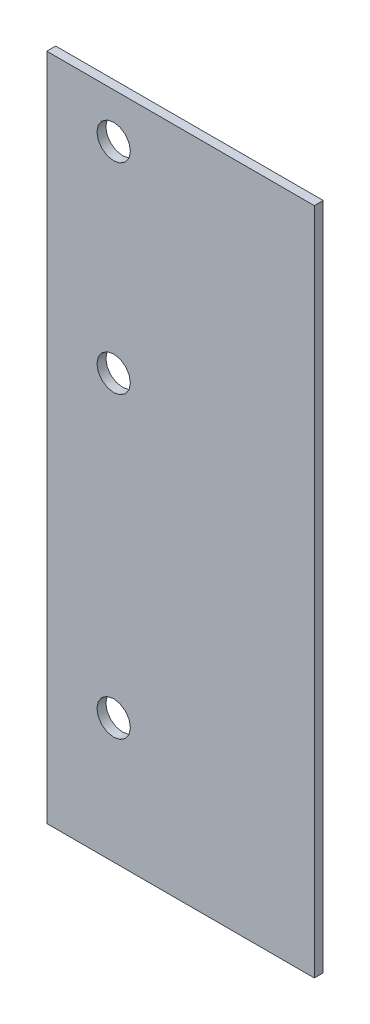
# Autodesk Inventor part: gabarito-suporte-motor-embaixo
Saved by Autodesk Inventor 2017 (Build 210142000, 142)
## iProperties
Created: 2018-08-18
Part Number: gabarito-suporte-motor-embaixo
Material: Wood (Oak)
Document SubType Name: Sheet Metal
Designer: Luiz Gustavo
Density: 0.76 g/cm^3
Sheet Metal Rule: Default_mm
Appearance: White Oak - Natural Medium Gloss
Author: Luiz Gustavo
Autodesk Inventor part; units mm, degrees
ref_plane "YZ Plane" through (0, 0, 0) normal (1, 0, 0) x (0, 1, 0)
ref_plane "XZ Plane" through (0, 0, 0) normal (0, 1, 0) x (-1, 0, 0)
ref_plane "XY Plane" through (0, 0, 0) normal (0, 0, 1) x (1, 0, 0)
sketch "Sketch1" plane through (0, 0, 0) normal (0, 0, 1) x (1, 0, 0)
  line L0 (16.1981, 153.4586) -> (16.9799, 152.4795) construction
  arc A0 (16.1981, 153.4586) -> (16.1981, 156.4471) centre (13, 154.9529) ccw construction
  line L1 (16.9799, 157.4262) -> (16.1981, 156.4471) construction
  arc A1 (16.9799, 157.4262) -> (15.4733, 158.9328) centre (16.1422, 158.0951) ccw construction
  line L2 (14.4942, 158.151) -> (15.4733, 158.9328) construction
  arc A2 (14.4942, 158.151) -> (11.5058, 158.151) centre (13, 154.9529) ccw construction
  line L3 (10.5267, 158.9328) -> (11.5058, 158.151) construction
  arc A3 (10.5267, 158.9328) -> (9.0201, 157.4262) centre (9.8578, 158.0951) ccw construction
  line L4 (9.8019, 156.4471) -> (9.0201, 157.4262) construction
  arc A4 (9.8019, 156.4471) -> (9.8019, 153.4586) centre (13, 154.9529) ccw construction
  line L5 (9.0201, 152.4795) -> (9.8019, 153.4586) construction
  arc A5 (9.0201, 152.4795) -> (10.5267, 150.9729) centre (9.8578, 151.8106) ccw construction
  line L6 (11.5058, 151.7547) -> (10.5267, 150.9729) construction
  arc A6 (11.5058, 151.7547) -> (14.4942, 151.7547) centre (13, 154.9529) ccw construction
  line L7 (15.4733, 150.9729) -> (14.4942, 151.7547) construction
  arc A7 (15.4733, 150.9729) -> (16.9799, 152.4795) centre (16.1422, 151.8106) ccw construction
  line L8 (26.6999, 145.0719) -> (26.6999, 142.2529) construction
  arc A8 (26.6999, 145.0719) -> (26.319, 145.4529) centre (26.319, 145.0719) ccw construction
  line L9 (22.88, 145.4529) -> (26.319, 145.4529) construction
  arc A9 (22.88, 145.4529) -> (22.5, 145.0729) centre (22.88, 145.0729) ccw construction
  line L10 (22.5, 141.6339) -> (22.5, 145.0729) construction
  arc A10 (22.5, 141.6339) -> (22.881, 141.2529) centre (22.881, 141.6339) ccw construction
  line L11 (25.7, 141.2529) -> (22.881, 141.2529) construction
  arc A11 (25.7, 141.2529) -> (26.6999, 142.2529) centre (25.7, 142.2529) ccw construction
  line L12 (-0.6999, 164.8338) -> (-0.6999, 167.6528) construction
  arc A12 (-0.6999, 164.8338) -> (-0.3189, 164.4528) centre (-0.3189, 164.8338) ccw construction
  line L13 (3.12, 164.4528) -> (-0.3189, 164.4528) construction
  arc A13 (3.12, 164.4528) -> (3.5, 164.8328) centre (3.12, 164.8328) ccw construction
  line L14 (3.5, 168.2718) -> (3.5, 164.8328) construction
  arc A14 (3.5, 168.2718) -> (3.119, 168.6528) centre (3.119, 168.2718) ccw construction
  line L15 (0.3001, 168.6528) -> (3.119, 168.6528) construction
  arc A15 (0.3001, 168.6528) -> (-0.6999, 167.6528) centre (0.3001, 167.6528) ccw construction
  line L16 (22.881, 168.6528) -> (25.7, 168.6528) construction
  arc A16 (22.881, 168.6528) -> (22.5, 168.2718) centre (22.881, 168.2718) ccw construction
  line L17 (22.5, 164.8328) -> (22.5, 168.2718) construction
  arc A17 (22.5, 164.8328) -> (22.88, 164.4528) centre (22.88, 164.8328) ccw construction
  line L18 (26.319, 164.4528) -> (22.88, 164.4528) construction
  arc A18 (26.319, 164.4528) -> (26.6999, 164.8338) centre (26.319, 164.8338) ccw construction
  line L19 (26.6999, 167.6528) -> (26.6999, 164.8338) construction
  arc A19 (26.6999, 167.6528) -> (25.7, 168.6528) centre (25.7, 167.6528) ccw construction
  line L20 (-0.3189, 145.4529) -> (3.12, 145.4529) construction
  arc A20 (-0.3189, 145.4529) -> (-0.6999, 145.0719) centre (-0.3189, 145.0719) ccw construction
  line L21 (-0.6999, 142.2529) -> (-0.6999, 145.0719) construction
  arc A21 (-0.6999, 142.2529) -> (0.3001, 141.2529) centre (0.3001, 142.2529) ccw construction
  line L22 (3.119, 141.2529) -> (0.3001, 141.2529) construction
  arc A22 (3.119, 141.2529) -> (3.5, 141.6339) centre (3.119, 141.6339) ccw construction
  line L23 (3.5, 145.0729) -> (3.5, 141.6339) construction
  arc A23 (3.5, 145.0729) -> (3.12, 145.4529) centre (3.12, 145.0729) ccw construction
  line L24 (8.5, 142.2104) -> (5.2675, 142.2104) construction
  arc A24 (9, 141.7104) -> (8.5, 142.2104) centre (8.5, 141.7104) ccw construction
  line L25 (9, 140.4529) -> (9, 141.7104) construction
  arc A25 (8.5, 139.9529) -> (9, 140.4529) centre (8.5, 140.4529) ccw construction
  line L26 (0.0001, 139.9529) -> (8.5, 139.9529) construction
  arc A26 (-1.9999, 141.9529) -> (0.0001, 139.9529) centre (0.0001, 141.9529) ccw construction
  line L27 (-1.9999, 150.4529) -> (-1.9999, 141.9529) construction
  arc A27 (-1.4999, 150.9529) -> (-1.9999, 150.4529) centre (-1.4999, 150.4529) ccw construction
  line L28 (-0.2425, 150.9529) -> (-1.4999, 150.9529) construction
  arc A28 (0.2575, 150.4529) -> (-0.2425, 150.9529) centre (-0.2425, 150.4529) ccw construction
  line L29 (0.2575, 147.2203) -> (0.2575, 150.4529) construction
  arc A29 (0.2575, 147.2203) -> (0.7572, 146.7029) centre (0.7572, 147.2029) ccw construction
  line L30 (2.7398, 146.7029) -> (0.7572, 146.7029) construction
  arc A30 (2.7398, 146.7029) -> (3.0934, 146.8493) centre (2.7398, 147.2029) ccw construction
  line L31 (7.0189, 150.7749) -> (3.0934, 146.8493) construction
  arc A31 (7.0189, 150.7749) -> (7.1653, 151.1284) centre (6.6653, 151.1284) ccw construction
  line L32 (7.1653, 154.0029) -> (7.1653, 151.1284) construction
  line L33 (7.6753, 154.9529) -> (7.1653, 154.0029) construction
  line L34 (7.1653, 155.9029) -> (7.6753, 154.9529) construction
  line L35 (7.1653, 158.7773) -> (7.1653, 155.9029) construction
  arc A32 (7.1653, 158.7773) -> (7.0189, 159.1309) centre (6.6653, 158.7773) ccw construction
  line L36 (3.0934, 163.0564) -> (7.0189, 159.1309) construction
  arc A33 (3.0934, 163.0564) -> (2.7398, 163.2028) centre (2.7398, 162.7028) ccw construction
  line L37 (0.7572, 163.2028) -> (2.7398, 163.2028) construction
  arc A34 (0.7572, 163.2028) -> (0.2575, 162.6854) centre (0.7572, 162.7028) ccw construction
  line L38 (0.2575, 159.4529) -> (0.2575, 162.6854) construction
  arc A35 (-0.2425, 158.9529) -> (0.2575, 159.4529) centre (-0.2425, 159.4529) ccw construction
  line L39 (-1.4999, 158.9529) -> (-0.2425, 158.9529) construction
  arc A36 (-1.9999, 159.4529) -> (-1.4999, 158.9529) centre (-1.4999, 159.4529) ccw construction
  line L40 (-1.9999, 167.9528) -> (-1.9999, 159.4529) construction
  arc A37 (0.0001, 169.9528) -> (-1.9999, 167.9528) centre (0.0001, 167.9528) ccw construction
  line L41 (8.5, 169.9528) -> (0.0001, 169.9528) construction
  arc A38 (9, 169.4528) -> (8.5, 169.9528) centre (8.5, 169.4528) ccw construction
  line L42 (9, 168.1953) -> (9, 169.4528) construction
  arc A39 (8.5, 167.6953) -> (9, 168.1953) centre (8.5, 168.1953) ccw construction
  line L43 (5.2675, 167.6953) -> (8.5, 167.6953) construction
  arc A40 (5.2675, 167.6953) -> (4.75, 167.1956) centre (5.25, 167.1956) ccw construction
  line L44 (4.75, 165.2131) -> (4.75, 167.1956) construction
  arc A41 (4.75, 165.2131) -> (4.8965, 164.8595) centre (5.25, 165.2131) ccw construction
  line L45 (8.822, 160.934) -> (4.8965, 164.8595) construction
  arc A42 (8.822, 160.934) -> (9.1756, 160.7875) centre (9.1756, 161.2875) ccw construction
  line L46 (12.1125, 160.7875) -> (9.1756, 160.7875) construction
  line L47 (13.0625, 160.2775) -> (12.1125, 160.7875) construction
  line L48 (14.0125, 160.7875) -> (13.0625, 160.2775) construction
  line L49 (16.8245, 160.7875) -> (14.0125, 160.7875) construction
  arc A43 (16.8245, 160.7875) -> (17.178, 160.934) centre (16.8245, 161.2875) ccw construction
  line L50 (21.1035, 164.8595) -> (17.178, 160.934) construction
  arc A44 (21.1035, 164.8595) -> (21.25, 165.2131) centre (20.75, 165.2131) ccw construction
  line L51 (21.25, 167.1956) -> (21.25, 165.2131) construction
  arc A45 (21.25, 167.1956) -> (20.7325, 167.6953) centre (20.75, 167.1956) ccw construction
  line L52 (17.5, 167.6953) -> (20.7325, 167.6953) construction
  arc A46 (17, 168.1953) -> (17.5, 167.6953) centre (17.5, 168.1953) ccw construction
  line L53 (17, 169.4528) -> (17, 168.1953) construction
  arc A47 (17.5, 169.9528) -> (17, 169.4528) centre (17.5, 169.4528) ccw construction
  line L54 (26, 169.9528) -> (17.5, 169.9528) construction
  arc A48 (27.9999, 167.9528) -> (26, 169.9528) centre (26, 167.9528) ccw construction
  line L55 (27.9999, 159.4529) -> (27.9999, 167.9528) construction
  arc A49 (27.4999, 158.9529) -> (27.9999, 159.4529) centre (27.4999, 159.4529) ccw construction
  line L56 (26.2425, 158.9529) -> (27.4999, 158.9529) construction
  arc A50 (25.7425, 159.4529) -> (26.2425, 158.9529) centre (26.2425, 159.4529) ccw construction
  line L57 (25.7425, 162.6854) -> (25.7425, 159.4529) construction
  arc A51 (25.7425, 162.6854) -> (25.2428, 163.2028) centre (25.2428, 162.7028) ccw construction
  line L58 (23.2602, 163.2028) -> (25.2428, 163.2028) construction
  arc A52 (23.2602, 163.2028) -> (22.9066, 163.0564) centre (23.2602, 162.7028) ccw construction
  line L59 (18.9811, 159.1309) -> (22.9066, 163.0564) construction
  arc A53 (18.9811, 159.1309) -> (18.8347, 158.7773) centre (19.3347, 158.7773) ccw construction
  line L60 (18.8347, 155.9029) -> (18.8347, 158.7773) construction
  line L61 (18.3247, 154.9529) -> (18.8347, 155.9029) construction
  line L62 (18.8347, 154.0029) -> (18.3247, 154.9529) construction
  line L63 (18.8347, 151.1284) -> (18.8347, 154.0029) construction
  arc A54 (18.8347, 151.1284) -> (18.9811, 150.7749) centre (19.3347, 151.1284) ccw construction
  line L64 (22.9066, 146.8493) -> (18.9811, 150.7749) construction
  arc A55 (22.9066, 146.8493) -> (23.2602, 146.7029) centre (23.2602, 147.2029) ccw construction
  line L65 (25.2428, 146.7029) -> (23.2602, 146.7029) construction
  arc A56 (25.2428, 146.7029) -> (25.7425, 147.2203) centre (25.2428, 147.2029) ccw construction
  line L66 (25.7425, 150.4529) -> (25.7425, 147.2203) construction
  arc A57 (26.2425, 150.9529) -> (25.7425, 150.4529) centre (26.2425, 150.4529) ccw construction
  line L67 (27.4999, 150.9529) -> (26.2425, 150.9529) construction
  arc A58 (27.9999, 150.4529) -> (27.4999, 150.9529) centre (27.4999, 150.4529) ccw construction
  line L68 (27.9999, 141.9529) -> (27.9999, 150.4529) construction
  arc A59 (26, 139.9529) -> (27.9999, 141.9529) centre (26, 141.9529) ccw construction
  line L69 (17.5, 139.9529) -> (26, 139.9529) construction
  arc A60 (17, 140.4529) -> (17.5, 139.9529) centre (17.5, 140.4529) ccw construction
  line L70 (17, 141.7104) -> (17, 140.4529) construction
  arc A61 (17.5, 142.2104) -> (17, 141.7104) centre (17.5, 141.7104) ccw construction
  line L71 (20.7325, 142.2104) -> (17.5, 142.2104) construction
  arc A62 (20.7325, 142.2104) -> (21.25, 142.7101) centre (20.75, 142.7101) ccw construction
  line L72 (21.25, 144.6927) -> (21.25, 142.7101) construction
  arc A63 (21.25, 144.6927) -> (21.1035, 145.0462) centre (20.75, 144.6927) ccw construction
  line L73 (17.178, 148.9717) -> (21.1035, 145.0462) construction
  arc A64 (17.178, 148.9717) -> (16.8245, 149.1182) centre (16.8245, 148.6182) ccw construction
  line L74 (14.0125, 149.1182) -> (16.8245, 149.1182) construction
  line L75 (13.0625, 149.6282) -> (14.0125, 149.1182) construction
  line L76 (12.1125, 149.1182) -> (13.0625, 149.6282) construction
  line L77 (9.1756, 149.1182) -> (12.1125, 149.1182) construction
  arc A65 (9.1756, 149.1182) -> (8.822, 148.9717) centre (9.1756, 148.6182) ccw construction
  line L78 (4.8965, 145.0462) -> (8.822, 148.9717) construction
  arc A66 (4.8965, 145.0462) -> (4.75, 144.6927) centre (5.25, 144.6927) ccw construction
  line L79 (4.75, 142.7101) -> (4.75, 144.6927) construction
  arc A67 (4.75, 142.7101) -> (5.2675, 142.2104) centre (5.25, 142.7101) ccw construction
  line L80 (16.1981, -1.4942) -> (16.9799, -2.4733) construction
  arc A68 (16.1981, -1.4942) -> (16.1981, 1.4942) centre (13, 0) ccw construction
  line L81 (16.9799, 2.4733) -> (16.1981, 1.4942) construction
  arc A69 (16.9799, 2.4733) -> (15.4733, 3.9799) centre (16.1422, 3.1422) ccw construction
  line L82 (14.4942, 3.1981) -> (15.4733, 3.9799) construction
  arc A70 (14.4942, 3.1981) -> (11.5058, 3.1981) centre (13, 0) ccw construction
  line L83 (10.5267, 3.9799) -> (11.5058, 3.1981) construction
  arc A71 (10.5267, 3.9799) -> (9.0201, 2.4733) centre (9.8578, 3.1422) ccw construction
  line L84 (9.8019, 1.4942) -> (9.0201, 2.4733) construction
  arc A72 (9.8019, 1.4942) -> (9.8019, -1.4942) centre (13, 0) ccw construction
  line L85 (9.0201, -2.4733) -> (9.8019, -1.4942) construction
  arc A73 (9.0201, -2.4733) -> (10.5267, -3.9799) centre (9.8578, -3.1422) ccw construction
  line L86 (11.5058, -3.1981) -> (10.5267, -3.9799) construction
  arc A74 (11.5058, -3.1981) -> (14.4942, -3.1981) centre (13, 0) ccw construction
  line L87 (15.4733, -3.9799) -> (14.4942, -3.1981) construction
  arc A75 (15.4733, -3.9799) -> (16.9799, -2.4733) centre (16.1422, -3.1422) ccw construction
  line L88 (26.6999, -9.881) -> (26.6999, -12.6999) construction
  arc A76 (26.6999, -9.881) -> (26.319, -9.5) centre (26.319, -9.881) ccw construction
  line L89 (22.88, -9.5) -> (26.319, -9.5) construction
  arc A77 (22.88, -9.5) -> (22.5, -9.88) centre (22.88, -9.88) ccw construction
  line L90 (22.5, -13.3189) -> (22.5, -9.88) construction
  arc A78 (22.5, -13.3189) -> (22.881, -13.6999) centre (22.881, -13.3189) ccw construction
  line L91 (25.7, -13.6999) -> (22.881, -13.6999) construction
  arc A79 (25.7, -13.6999) -> (26.6999, -12.6999) centre (25.7, -12.6999) ccw construction
  line L92 (-0.6999, 9.881) -> (-0.6999, 12.6999) construction
  arc A80 (-0.6999, 9.881) -> (-0.3189, 9.5) centre (-0.3189, 9.881) ccw construction
  line L93 (3.12, 9.5) -> (-0.3189, 9.5) construction
  arc A81 (3.12, 9.5) -> (3.5, 9.88) centre (3.12, 9.88) ccw construction
  line L94 (3.5, 13.3189) -> (3.5, 9.88) construction
  arc A82 (3.5, 13.3189) -> (3.119, 13.6999) centre (3.119, 13.3189) ccw construction
  line L95 (0.3001, 13.6999) -> (3.119, 13.6999) construction
  arc A83 (0.3001, 13.6999) -> (-0.6999, 12.6999) centre (0.3001, 12.6999) ccw construction
  line L96 (22.881, 13.6999) -> (25.7, 13.6999) construction
  arc A84 (22.881, 13.6999) -> (22.5, 13.3189) centre (22.881, 13.3189) ccw construction
  line L97 (22.5, 9.88) -> (22.5, 13.3189) construction
  arc A85 (22.5, 9.88) -> (22.88, 9.5) centre (22.88, 9.88) ccw construction
  line L98 (26.319, 9.5) -> (22.88, 9.5) construction
  arc A86 (26.319, 9.5) -> (26.6999, 9.881) centre (26.319, 9.881) ccw construction
  line L99 (26.6999, 12.6999) -> (26.6999, 9.881) construction
  arc A87 (26.6999, 12.6999) -> (25.7, 13.6999) centre (25.7, 12.6999) ccw construction
  line L100 (-0.3189, -9.5) -> (3.12, -9.5) construction
  arc A88 (-0.3189, -9.5) -> (-0.6999, -9.881) centre (-0.3189, -9.881) ccw construction
  line L101 (-0.6999, -12.6999) -> (-0.6999, -9.881) construction
  arc A89 (-0.6999, -12.6999) -> (0.3001, -13.6999) centre (0.3001, -12.6999) ccw construction
  line L102 (3.119, -13.6999) -> (0.3001, -13.6999) construction
  arc A90 (3.119, -13.6999) -> (3.5, -13.3189) centre (3.119, -13.3189) ccw construction
  line L103 (3.5, -9.88) -> (3.5, -13.3189) construction
  arc A91 (3.5, -9.88) -> (3.12, -9.5) centre (3.12, -9.88) ccw construction
  line L104 (8.5, -12.7425) -> (5.2675, -12.7425) construction
  arc A92 (9, -13.2425) -> (8.5, -12.7425) centre (8.5, -13.2425) ccw construction
  line L105 (9, -14.4999) -> (9, -13.2425) construction
  arc A93 (8.5, -14.9999) -> (9, -14.4999) centre (8.5, -14.4999) ccw construction
  line L106 (0.0001, -14.9999) -> (8.5, -14.9999) construction
  arc A94 (-1.9999, -12.9999) -> (0.0001, -14.9999) centre (0.0001, -12.9999) ccw construction
  line L107 (-1.9999, -4.5) -> (-1.9999, -12.9999) construction
  arc A95 (-1.4999, -4) -> (-1.9999, -4.5) centre (-1.4999, -4.5) ccw construction
  line L108 (-0.2425, -4) -> (-1.4999, -4) construction
  arc A96 (0.2575, -4.5) -> (-0.2425, -4) centre (-0.2425, -4.5) ccw construction
  line L109 (0.2575, -7.7325) -> (0.2575, -4.5) construction
  arc A97 (0.2575, -7.7325) -> (0.7572, -8.25) centre (0.7572, -7.75) ccw construction
  line L110 (2.7398, -8.25) -> (0.7572, -8.25) construction
  arc A98 (2.7398, -8.25) -> (3.0934, -8.1035) centre (2.7398, -7.75) ccw construction
  line L111 (7.0189, -4.178) -> (3.0934, -8.1035) construction
  arc A99 (7.0189, -4.178) -> (7.1653, -3.8245) centre (6.6653, -3.8245) ccw construction
  line L112 (7.1653, -0.95) -> (7.1653, -3.8245) construction
  line L113 (7.6753, 0) -> (7.1653, -0.95) construction
  line L114 (7.1653, 0.95) -> (7.6753, 0) construction
  line L115 (7.1653, 3.8245) -> (7.1653, 0.95) construction
  arc A100 (7.1653, 3.8245) -> (7.0189, 4.178) centre (6.6653, 3.8245) ccw construction
  line L116 (3.0934, 8.1035) -> (7.0189, 4.178) construction
  arc A101 (3.0934, 8.1035) -> (2.7398, 8.25) centre (2.7398, 7.75) ccw construction
  line L117 (0.7572, 8.25) -> (2.7398, 8.25) construction
  arc A102 (0.7572, 8.25) -> (0.2575, 7.7325) centre (0.7572, 7.75) ccw construction
  line L118 (0.2575, 4.5) -> (0.2575, 7.7325) construction
  arc A103 (-0.2425, 4) -> (0.2575, 4.5) centre (-0.2425, 4.5) ccw construction
  line L119 (-1.4999, 4) -> (-0.2425, 4) construction
  arc A104 (-1.9999, 4.5) -> (-1.4999, 4) centre (-1.4999, 4.5) ccw construction
  line L120 (-1.9999, 12.9999) -> (-1.9999, 4.5) construction
  arc A105 (0.0001, 14.9999) -> (-1.9999, 12.9999) centre (0.0001, 12.9999) ccw construction
  line L121 (8.5, 14.9999) -> (0.0001, 14.9999) construction
  arc A106 (9, 14.4999) -> (8.5, 14.9999) centre (8.5, 14.4999) ccw construction
  line L122 (9, 13.2425) -> (9, 14.4999) construction
  arc A107 (8.5, 12.7425) -> (9, 13.2425) centre (8.5, 13.2425) ccw construction
  line L123 (5.2675, 12.7425) -> (8.5, 12.7425) construction
  arc A108 (5.2675, 12.7425) -> (4.75, 12.2428) centre (5.25, 12.2428) ccw construction
  line L124 (4.75, 10.2602) -> (4.75, 12.2428) construction
  arc A109 (4.75, 10.2602) -> (4.8965, 9.9066) centre (5.25, 10.2602) ccw construction
  line L125 (8.822, 5.9811) -> (4.8965, 9.9066) construction
  arc A110 (8.822, 5.9811) -> (9.1756, 5.8347) centre (9.1756, 6.3347) ccw construction
  line L126 (12.1125, 5.8347) -> (9.1756, 5.8347) construction
  line L127 (13.0625, 5.3247) -> (12.1125, 5.8347) construction
  line L128 (14.0125, 5.8347) -> (13.0625, 5.3247) construction
  line L129 (16.8245, 5.8347) -> (14.0125, 5.8347) construction
  arc A111 (16.8245, 5.8347) -> (17.178, 5.9811) centre (16.8245, 6.3347) ccw construction
  line L130 (21.1035, 9.9066) -> (17.178, 5.9811) construction
  arc A112 (21.1035, 9.9066) -> (21.25, 10.2602) centre (20.75, 10.2602) ccw construction
  line L131 (21.25, 12.2428) -> (21.25, 10.2602) construction
  arc A113 (21.25, 12.2428) -> (20.7325, 12.7425) centre (20.75, 12.2428) ccw construction
  line L132 (17.5, 12.7425) -> (20.7325, 12.7425) construction
  arc A114 (17, 13.2425) -> (17.5, 12.7425) centre (17.5, 13.2425) ccw construction
  line L133 (17, 14.4999) -> (17, 13.2425) construction
  arc A115 (17.5, 14.9999) -> (17, 14.4999) centre (17.5, 14.4999) ccw construction
  line L134 (26, 14.9999) -> (17.5, 14.9999) construction
  arc A116 (27.9999, 12.9999) -> (26, 14.9999) centre (26, 12.9999) ccw construction
  line L135 (27.9999, 4.5) -> (27.9999, 12.9999) construction
  arc A117 (27.4999, 4) -> (27.9999, 4.5) centre (27.4999, 4.5) ccw construction
  line L136 (26.2425, 4) -> (27.4999, 4) construction
  arc A118 (25.7425, 4.5) -> (26.2425, 4) centre (26.2425, 4.5) ccw construction
  line L137 (25.7425, 7.7325) -> (25.7425, 4.5) construction
  arc A119 (25.7425, 7.7325) -> (25.2428, 8.25) centre (25.2428, 7.75) ccw construction
  line L138 (23.2602, 8.25) -> (25.2428, 8.25) construction
  arc A120 (23.2602, 8.25) -> (22.9066, 8.1035) centre (23.2602, 7.75) ccw construction
  line L139 (18.9811, 4.178) -> (22.9066, 8.1035) construction
  arc A121 (18.9811, 4.178) -> (18.8347, 3.8245) centre (19.3347, 3.8245) ccw construction
  line L140 (18.8347, 0.95) -> (18.8347, 3.8245) construction
  line L141 (18.3247, 0) -> (18.8347, 0.95) construction
  line L142 (18.8347, -0.95) -> (18.3247, 0) construction
  line L143 (18.8347, -3.8245) -> (18.8347, -0.95) construction
  arc A122 (18.8347, -3.8245) -> (18.9811, -4.178) centre (19.3347, -3.8245) ccw construction
  line L144 (22.9066, -8.1035) -> (18.9811, -4.178) construction
  arc A123 (22.9066, -8.1035) -> (23.2602, -8.25) centre (23.2602, -7.75) ccw construction
  line L145 (25.2428, -8.25) -> (23.2602, -8.25) construction
  arc A124 (25.2428, -8.25) -> (25.7425, -7.7325) centre (25.2428, -7.75) ccw construction
  line L146 (25.7425, -4.5) -> (25.7425, -7.7325) construction
  arc A125 (26.2425, -4) -> (25.7425, -4.5) centre (26.2425, -4.5) ccw construction
  line L147 (27.4999, -4) -> (26.2425, -4) construction
  arc A126 (27.9999, -4.5) -> (27.4999, -4) centre (27.4999, -4.5) ccw construction
  line L148 (27.9999, -12.9999) -> (27.9999, -4.5) construction
  arc A127 (26, -14.9999) -> (27.9999, -12.9999) centre (26, -12.9999) ccw construction
  line L149 (17.5, -14.9999) -> (26, -14.9999) construction
  arc A128 (17, -14.4999) -> (17.5, -14.9999) centre (17.5, -14.4999) ccw construction
  line L150 (17, -13.2425) -> (17, -14.4999) construction
  arc A129 (17.5, -12.7425) -> (17, -13.2425) centre (17.5, -13.2425) ccw construction
  line L151 (20.7325, -12.7425) -> (17.5, -12.7425) construction
  arc A130 (20.7325, -12.7425) -> (21.25, -12.2428) centre (20.75, -12.2428) ccw construction
  line L152 (21.25, -10.2602) -> (21.25, -12.2428) construction
  arc A131 (21.25, -10.2602) -> (21.1035, -9.9066) centre (20.75, -10.2602) ccw construction
  line L153 (17.178, -5.9811) -> (21.1035, -9.9066) construction
  arc A132 (17.178, -5.9811) -> (16.8245, -5.8347) centre (16.8245, -6.3347) ccw construction
  line L154 (14.0125, -5.8347) -> (16.8245, -5.8347) construction
  line L155 (13.0625, -5.3247) -> (14.0125, -5.8347) construction
  line L156 (12.1125, -5.8347) -> (13.0625, -5.3247) construction
  line L157 (9.1756, -5.8347) -> (12.1125, -5.8347) construction
  arc A133 (9.1756, -5.8347) -> (8.822, -5.9811) centre (9.1756, -6.3347) ccw construction
  line L158 (4.8965, -9.9066) -> (8.822, -5.9811) construction
  arc A134 (4.8965, -9.9066) -> (4.75, -10.2602) centre (5.25, -10.2602) ccw construction
  line L159 (4.75, -12.2428) -> (4.75, -10.2602) construction
  arc A135 (4.75, -12.2428) -> (5.2675, -12.7425) centre (5.25, -12.2428) ccw construction
  line L160 (8.5, 122.6953) -> (5.2675, 122.6953) construction
  arc A136 (5.2675, 122.6953) -> (4.75, 122.1956) centre (5.25, 122.1956) ccw construction
  line L161 (4.75, 122.1956) -> (4.75, 120.2131) construction
  arc A137 (4.75, 120.2131) -> (4.8965, 119.8595) centre (5.25, 120.2131) ccw construction
  line L162 (4.8965, 119.8595) -> (8.822, 115.934) construction
  arc A138 (8.822, 115.934) -> (9.1756, 115.7875) centre (9.1756, 116.2875) ccw construction
  line L163 (9.1756, 115.7875) -> (12.1125, 115.7875) construction
  line L164 (12.1125, 115.7875) -> (13.0625, 115.2775) construction
  line L165 (13.0625, 115.2775) -> (14.0125, 115.7875) construction
  line L166 (14.0125, 115.7875) -> (16.8245, 115.7875) construction
  arc A139 (16.8245, 115.7875) -> (17.178, 115.934) centre (16.8245, 116.2875) ccw construction
  line L167 (17.178, 115.934) -> (21.1035, 119.8595) construction
  arc A140 (21.1035, 119.8595) -> (21.25, 120.2131) centre (20.75, 120.2131) ccw construction
  line L168 (21.25, 120.2131) -> (21.25, 122.1956) construction
  arc A141 (21.25, 122.1956) -> (20.7325, 122.6953) centre (20.75, 122.1956) ccw construction
  line L169 (20.7325, 122.6953) -> (17.5, 122.6953) construction
  arc A142 (17, 123.1953) -> (17.5, 122.6953) centre (17.5, 123.1953) ccw construction
  line L170 (17, 123.1953) -> (17, 124.4528) construction
  arc A143 (17.5, 124.9528) -> (17, 124.4528) centre (17.5, 124.4528) ccw construction
  line L171 (17.5, 124.9528) -> (26, 124.9528) construction
  arc A144 (27.9999, 122.9528) -> (26, 124.9528) centre (26, 122.9528) ccw construction
  line L172 (27.9999, 122.9528) -> (27.9999, 114.4529) construction
  arc A145 (27.4999, 113.9529) -> (27.9999, 114.4529) centre (27.4999, 114.4529) ccw construction
  line L173 (27.4999, 113.9529) -> (26.2425, 113.9529) construction
  arc A146 (25.7425, 114.4529) -> (26.2425, 113.9529) centre (26.2425, 114.4529) ccw construction
  line L174 (25.7425, 114.4529) -> (25.7425, 117.6854) construction
  arc A147 (25.7425, 117.6854) -> (25.2428, 118.2028) centre (25.2428, 117.7028) ccw construction
  line L175 (25.2428, 118.2028) -> (23.2602, 118.2028) construction
  arc A148 (23.2602, 118.2028) -> (22.9066, 118.0564) centre (23.2602, 117.7028) ccw construction
  line L176 (22.9066, 118.0564) -> (18.9811, 114.1309) construction
  arc A149 (18.9811, 114.1309) -> (18.8347, 113.7773) centre (19.3347, 113.7773) ccw construction
  line L177 (18.8347, 113.7773) -> (18.8347, 110.9029) construction
  line L178 (18.8347, 110.9029) -> (18.3247, 109.9529) construction
  line L179 (18.3247, 109.9529) -> (18.8347, 109.0029) construction
  line L180 (18.8347, 109.0029) -> (18.8347, 106.1284) construction
  arc A150 (18.8347, 106.1284) -> (18.9811, 105.7749) centre (19.3347, 106.1284) ccw construction
  line L181 (18.9811, 105.7749) -> (22.9066, 101.8493) construction
  arc A151 (22.9066, 101.8493) -> (23.2602, 101.7029) centre (23.2602, 102.2029) ccw construction
  line L182 (23.2602, 101.7029) -> (25.2428, 101.7029) construction
  arc A152 (25.2428, 101.7029) -> (25.7425, 102.2203) centre (25.2428, 102.2029) ccw construction
  line L183 (25.7425, 102.2203) -> (25.7425, 105.4529) construction
  arc A153 (26.2425, 105.9529) -> (25.7425, 105.4529) centre (26.2425, 105.4529) ccw construction
  line L184 (26.2425, 105.9529) -> (27.4999, 105.9529) construction
  arc A154 (27.9999, 105.4529) -> (27.4999, 105.9529) centre (27.4999, 105.4529) ccw construction
  line L185 (27.9999, 105.4529) -> (27.9999, 96.9529) construction
  arc A155 (26, 94.9529) -> (27.9999, 96.9529) centre (26, 96.9529) ccw construction
  line L186 (26, 94.9529) -> (17.5, 94.9529) construction
  arc A156 (17, 95.4529) -> (17.5, 94.9529) centre (17.5, 95.4529) ccw construction
  line L187 (17, 95.4529) -> (17, 96.7104) construction
  arc A157 (17.5, 97.2104) -> (17, 96.7104) centre (17.5, 96.7104) ccw construction
  line L188 (17.5, 97.2104) -> (20.7325, 97.2104) construction
  arc A158 (20.7325, 97.2104) -> (21.25, 97.7101) centre (20.75, 97.7101) ccw construction
  line L189 (21.25, 97.7101) -> (21.25, 99.6927) construction
  arc A159 (21.25, 99.6927) -> (21.1035, 100.0462) centre (20.75, 99.6927) ccw construction
  line L190 (21.1035, 100.0462) -> (17.178, 103.9717) construction
  arc A160 (17.178, 103.9717) -> (16.8245, 104.1182) centre (16.8245, 103.6182) ccw construction
  line L191 (16.8245, 104.1182) -> (14.0125, 104.1182) construction
  line L192 (14.0125, 104.1182) -> (13.0625, 104.6282) construction
  line L193 (13.0625, 104.6282) -> (12.1125, 104.1182) construction
  line L194 (12.1125, 104.1182) -> (9.1756, 104.1182) construction
  arc A161 (9.1756, 104.1182) -> (8.822, 103.9717) centre (9.1756, 103.6182) ccw construction
  line L195 (8.822, 103.9717) -> (4.8965, 100.0462) construction
  arc A162 (4.8965, 100.0462) -> (4.75, 99.6927) centre (5.25, 99.6927) ccw construction
  line L196 (4.75, 99.6927) -> (4.75, 97.7101) construction
  arc A163 (4.75, 97.7101) -> (5.2675, 97.2104) centre (5.25, 97.7101) ccw construction
  line L197 (5.2675, 97.2104) -> (8.5, 97.2104) construction
  arc A164 (9, 96.7104) -> (8.5, 97.2104) centre (8.5, 96.7104) ccw construction
  line L198 (9, 96.7104) -> (9, 95.4529) construction
  arc A165 (8.5, 94.9529) -> (9, 95.4529) centre (8.5, 95.4529) ccw construction
  line L199 (8.5, 94.9529) -> (0.0001, 94.9529) construction
  arc A166 (-1.9999, 96.9529) -> (0.0001, 94.9529) centre (0.0001, 96.9529) ccw construction
  line L200 (-1.9999, 96.9529) -> (-1.9999, 105.4529) construction
  arc A167 (-1.4999, 105.9529) -> (-1.9999, 105.4529) centre (-1.4999, 105.4529) ccw construction
  line L201 (-1.4999, 105.9529) -> (-0.2425, 105.9529) construction
  arc A168 (0.2575, 105.4529) -> (-0.2425, 105.9529) centre (-0.2425, 105.4529) ccw construction
  line L202 (0.2575, 105.4529) -> (0.2575, 102.2203) construction
  arc A169 (0.2575, 102.2203) -> (0.7572, 101.7029) centre (0.7572, 102.2029) ccw construction
  line L203 (0.7572, 101.7029) -> (2.7398, 101.7029) construction
  arc A170 (2.7398, 101.7029) -> (3.0934, 101.8493) centre (2.7398, 102.2029) ccw construction
  line L204 (3.0934, 101.8493) -> (7.0189, 105.7749) construction
  arc A171 (7.0189, 105.7749) -> (7.1653, 106.1284) centre (6.6653, 106.1284) ccw construction
  line L205 (7.1653, 106.1284) -> (7.1653, 109.0029) construction
  line L206 (7.1653, 109.0029) -> (7.6753, 109.9529) construction
  line L207 (7.6753, 109.9529) -> (7.1653, 110.9029) construction
  line L208 (7.1653, 110.9029) -> (7.1653, 113.7773) construction
  arc A172 (7.1653, 113.7773) -> (7.0189, 114.1309) centre (6.6653, 113.7773) ccw construction
  line L209 (7.0189, 114.1309) -> (3.0934, 118.0564) construction
  arc A173 (3.0934, 118.0564) -> (2.7398, 118.2028) centre (2.7398, 117.7028) ccw construction
  line L210 (2.7398, 118.2028) -> (0.7572, 118.2028) construction
  arc A174 (0.7572, 118.2028) -> (0.2575, 117.6854) centre (0.7572, 117.7028) ccw construction
  line L211 (0.2575, 117.6854) -> (0.2575, 114.4529) construction
  arc A175 (-0.2425, 113.9529) -> (0.2575, 114.4529) centre (-0.2425, 114.4529) ccw construction
  line L212 (-0.2425, 113.9529) -> (-1.4999, 113.9529) construction
  arc A176 (-1.9999, 114.4529) -> (-1.4999, 113.9529) centre (-1.4999, 114.4529) ccw construction
  line L213 (-1.9999, 114.4529) -> (-1.9999, 122.9528) construction
  arc A177 (0.0001, 124.9528) -> (-1.9999, 122.9528) centre (0.0001, 122.9528) ccw construction
  line L214 (0.0001, 124.9528) -> (8.5, 124.9528) construction
  arc A178 (9, 124.4528) -> (8.5, 124.9528) centre (8.5, 124.4528) ccw construction
  line L215 (9, 124.4528) -> (9, 123.1953) construction
  arc A179 (8.5, 122.6953) -> (9, 123.1953) centre (8.5, 123.1953) ccw construction
  line L216 (16.1981, 44.4942) -> (16.9799, 45.4733) construction
  arc A180 (16.9799, 45.4733) -> (15.4733, 46.9799) centre (16.1422, 46.1422) ccw construction
  line L217 (15.4733, 46.9799) -> (14.4942, 46.1981) construction
  arc A181 (14.4942, 46.1981) -> (11.5058, 46.1981) centre (13, 43) ccw construction
  line L218 (11.5058, 46.1981) -> (10.5267, 46.9799) construction
  arc A182 (10.5267, 46.9799) -> (9.0201, 45.4733) centre (9.8578, 46.1422) ccw construction
  line L219 (9.0201, 45.4733) -> (9.8019, 44.4942) construction
  arc A183 (9.8019, 44.4942) -> (9.8019, 41.5058) centre (13, 43) ccw construction
  line L220 (9.8019, 41.5058) -> (9.0201, 40.5267) construction
  arc A184 (9.0201, 40.5267) -> (10.5267, 39.0201) centre (9.8578, 39.8578) ccw construction
  line L221 (10.5267, 39.0201) -> (11.5058, 39.8019) construction
  arc A185 (11.5058, 39.8019) -> (14.4942, 39.8019) centre (13, 43) ccw construction
  line L222 (14.4942, 39.8019) -> (15.4733, 39.0201) construction
  arc A186 (15.4733, 39.0201) -> (16.9799, 40.5267) centre (16.1422, 39.8578) ccw construction
  line L223 (16.9799, 40.5267) -> (16.1981, 41.5058) construction
  arc A187 (16.1981, 41.5058) -> (16.1981, 44.4942) centre (13, 43) ccw construction
  line L224 (26.6999, 52.881) -> (26.6999, 55.6999) construction
  arc A188 (26.6999, 55.6999) -> (25.7, 56.6999) centre (25.7, 55.6999) ccw construction
  line L225 (25.7, 56.6999) -> (22.881, 56.6999) construction
  arc A189 (22.881, 56.6999) -> (22.5, 56.3189) centre (22.881, 56.3189) ccw construction
  line L226 (22.5, 56.3189) -> (22.5, 52.88) construction
  arc A190 (22.5, 52.88) -> (22.88, 52.5) centre (22.88, 52.88) ccw construction
  line L227 (22.88, 52.5) -> (26.319, 52.5) construction
  arc A191 (26.319, 52.5) -> (26.6999, 52.881) centre (26.319, 52.881) ccw construction
  line L228 (-0.6999, 33.119) -> (-0.6999, 30.3001) construction
  arc A192 (-0.6999, 30.3001) -> (0.3001, 29.3001) centre (0.3001, 30.3001) ccw construction
  line L229 (0.3001, 29.3001) -> (3.119, 29.3001) construction
  arc A193 (3.119, 29.3001) -> (3.5, 29.6811) centre (3.119, 29.6811) ccw construction
  line L230 (3.5, 29.6811) -> (3.5, 33.12) construction
  arc A194 (3.5, 33.12) -> (3.12, 33.5) centre (3.12, 33.12) ccw construction
  line L231 (3.12, 33.5) -> (-0.3189, 33.5) construction
  arc A195 (-0.3189, 33.5) -> (-0.6999, 33.119) centre (-0.3189, 33.119) ccw construction
  line L232 (22.881, 29.3001) -> (25.7, 29.3001) construction
  arc A196 (25.7, 29.3001) -> (26.6999, 30.3001) centre (25.7, 30.3001) ccw construction
  line L233 (26.6999, 30.3001) -> (26.6999, 33.119) construction
  arc A197 (26.6999, 33.119) -> (26.319, 33.5) centre (26.319, 33.119) ccw construction
  line L234 (26.319, 33.5) -> (22.88, 33.5) construction
  arc A198 (22.88, 33.5) -> (22.5, 33.12) centre (22.88, 33.12) ccw construction
  line L235 (22.5, 33.12) -> (22.5, 29.6811) construction
  arc A199 (22.5, 29.6811) -> (22.881, 29.3001) centre (22.881, 29.6811) ccw construction
  line L236 (-0.3189, 52.5) -> (3.12, 52.5) construction
  arc A200 (3.12, 52.5) -> (3.5, 52.88) centre (3.12, 52.88) ccw construction
  line L237 (3.5, 52.88) -> (3.5, 56.3189) construction
  arc A201 (3.5, 56.3189) -> (3.119, 56.6999) centre (3.119, 56.3189) ccw construction
  line L238 (3.119, 56.6999) -> (0.3001, 56.6999) construction
  arc A202 (0.3001, 56.6999) -> (-0.6999, 55.6999) centre (0.3001, 55.6999) ccw construction
  line L239 (-0.6999, 55.6999) -> (-0.6999, 52.881) construction
  arc A203 (-0.6999, 52.881) -> (-0.3189, 52.5) centre (-0.3189, 52.881) ccw construction
  line L240 (8.5, 55.7425) -> (5.2675, 55.7425) construction
  arc A204 (5.2675, 55.7425) -> (4.75, 55.2428) centre (5.25, 55.2428) ccw construction
  line L241 (4.75, 55.2428) -> (4.75, 53.2602) construction
  arc A205 (4.75, 53.2602) -> (4.8965, 52.9066) centre (5.25, 53.2602) ccw construction
  line L242 (4.8965, 52.9066) -> (8.822, 48.9811) construction
  arc A206 (8.822, 48.9811) -> (9.1756, 48.8347) centre (9.1756, 49.3347) ccw construction
  line L243 (9.1756, 48.8347) -> (12.1125, 48.8347) construction
  line L244 (12.1125, 48.8347) -> (13.0625, 48.3247) construction
  line L245 (13.0625, 48.3247) -> (14.0125, 48.8347) construction
  line L246 (14.0125, 48.8347) -> (16.8245, 48.8347) construction
  arc A207 (16.8245, 48.8347) -> (17.178, 48.9811) centre (16.8245, 49.3347) ccw construction
  line L247 (17.178, 48.9811) -> (21.1035, 52.9066) construction
  arc A208 (21.1035, 52.9066) -> (21.25, 53.2602) centre (20.75, 53.2602) ccw construction
  line L248 (21.25, 53.2602) -> (21.25, 55.2428) construction
  arc A209 (21.25, 55.2428) -> (20.7325, 55.7425) centre (20.75, 55.2428) ccw construction
  line L249 (20.7325, 55.7425) -> (17.5, 55.7425) construction
  arc A210 (17, 56.2425) -> (17.5, 55.7425) centre (17.5, 56.2425) ccw construction
  line L250 (17, 56.2425) -> (17, 57.4999) construction
  arc A211 (17.5, 57.9999) -> (17, 57.4999) centre (17.5, 57.4999) ccw construction
  line L251 (17.5, 57.9999) -> (26, 57.9999) construction
  arc A212 (27.9999, 55.9999) -> (26, 57.9999) centre (26, 55.9999) ccw construction
  line L252 (27.9999, 55.9999) -> (27.9999, 47.5) construction
  arc A213 (27.4999, 47) -> (27.9999, 47.5) centre (27.4999, 47.5) ccw construction
  line L253 (27.4999, 47) -> (26.2425, 47) construction
  arc A214 (25.7425, 47.5) -> (26.2425, 47) centre (26.2425, 47.5) ccw construction
  line L254 (25.7425, 47.5) -> (25.7425, 50.7325) construction
  arc A215 (25.7425, 50.7325) -> (25.2428, 51.25) centre (25.2428, 50.75) ccw construction
  line L255 (25.2428, 51.25) -> (23.2602, 51.25) construction
  arc A216 (23.2602, 51.25) -> (22.9066, 51.1035) centre (23.2602, 50.75) ccw construction
  line L256 (22.9066, 51.1035) -> (18.9811, 47.178) construction
  arc A217 (18.9811, 47.178) -> (18.8347, 46.8245) centre (19.3347, 46.8245) ccw construction
  line L257 (18.8347, 46.8245) -> (18.8347, 43.95) construction
  line L258 (18.8347, 43.95) -> (18.3247, 43) construction
  line L259 (18.3247, 43) -> (18.8347, 42.05) construction
  line L260 (18.8347, 42.05) -> (18.8347, 39.1755) construction
  arc A218 (18.8347, 39.1755) -> (18.9811, 38.822) centre (19.3347, 39.1755) ccw construction
  line L261 (18.9811, 38.822) -> (22.9066, 34.8965) construction
  arc A219 (22.9066, 34.8965) -> (23.2602, 34.75) centre (23.2602, 35.25) ccw construction
  line L262 (23.2602, 34.75) -> (25.2428, 34.75) construction
  arc A220 (25.2428, 34.75) -> (25.7425, 35.2675) centre (25.2428, 35.25) ccw construction
  line L263 (25.7425, 35.2675) -> (25.7425, 38.5) construction
  arc A221 (26.2425, 39) -> (25.7425, 38.5) centre (26.2425, 38.5) ccw construction
  line L264 (26.2425, 39) -> (27.4999, 39) construction
  arc A222 (27.9999, 38.5) -> (27.4999, 39) centre (27.4999, 38.5) ccw construction
  line L265 (27.9999, 38.5) -> (27.9999, 30.0001) construction
  arc A223 (26, 28.0001) -> (27.9999, 30.0001) centre (26, 30.0001) ccw construction
  line L266 (26, 28.0001) -> (17.5, 28.0001) construction
  arc A224 (17, 28.5001) -> (17.5, 28.0001) centre (17.5, 28.5001) ccw construction
  line L267 (17, 28.5001) -> (17, 29.7575) construction
  arc A225 (17.5, 30.2575) -> (17, 29.7575) centre (17.5, 29.7575) ccw construction
  line L268 (17.5, 30.2575) -> (20.7325, 30.2575) construction
  arc A226 (20.7325, 30.2575) -> (21.25, 30.7572) centre (20.75, 30.7572) ccw construction
  line L269 (21.25, 30.7572) -> (21.25, 32.7398) construction
  arc A227 (21.25, 32.7398) -> (21.1035, 33.0934) centre (20.75, 32.7398) ccw construction
  line L270 (21.1035, 33.0934) -> (17.178, 37.0189) construction
  arc A228 (17.178, 37.0189) -> (16.8245, 37.1653) centre (16.8245, 36.6653) ccw construction
  line L271 (16.8245, 37.1653) -> (14.0125, 37.1653) construction
  line L272 (14.0125, 37.1653) -> (13.0625, 37.6753) construction
  line L273 (13.0625, 37.6753) -> (12.1125, 37.1653) construction
  line L274 (12.1125, 37.1653) -> (9.1756, 37.1653) construction
  arc A229 (9.1756, 37.1653) -> (8.822, 37.0189) centre (9.1756, 36.6653) ccw construction
  line L275 (8.822, 37.0189) -> (4.8965, 33.0934) construction
  arc A230 (4.8965, 33.0934) -> (4.75, 32.7398) centre (5.25, 32.7398) ccw construction
  line L276 (4.75, 32.7398) -> (4.75, 30.7572) construction
  arc A231 (4.75, 30.7572) -> (5.2675, 30.2575) centre (5.25, 30.7572) ccw construction
  line L277 (5.2675, 30.2575) -> (8.5, 30.2575) construction
  arc A232 (9, 29.7575) -> (8.5, 30.2575) centre (8.5, 29.7575) ccw construction
  line L278 (9, 29.7575) -> (9, 28.5001) construction
  arc A233 (8.5, 28.0001) -> (9, 28.5001) centre (8.5, 28.5001) ccw construction
  line L279 (8.5, 28.0001) -> (0.0001, 28.0001) construction
  arc A234 (-1.9999, 30.0001) -> (0.0001, 28.0001) centre (0.0001, 30.0001) ccw construction
  line L280 (-1.9999, 30.0001) -> (-1.9999, 38.5) construction
  arc A235 (-1.4999, 39) -> (-1.9999, 38.5) centre (-1.4999, 38.5) ccw construction
  line L281 (-1.4999, 39) -> (-0.2425, 39) construction
  arc A236 (0.2575, 38.5) -> (-0.2425, 39) centre (-0.2425, 38.5) ccw construction
  line L282 (0.2575, 38.5) -> (0.2575, 35.2675) construction
  arc A237 (0.2575, 35.2675) -> (0.7572, 34.75) centre (0.7572, 35.25) ccw construction
  line L283 (0.7572, 34.75) -> (2.7398, 34.75) construction
  arc A238 (2.7398, 34.75) -> (3.0934, 34.8965) centre (2.7398, 35.25) ccw construction
  line L284 (3.0934, 34.8965) -> (7.0189, 38.822) construction
  arc A239 (7.0189, 38.822) -> (7.1653, 39.1755) centre (6.6653, 39.1755) ccw construction
  line L285 (7.1653, 39.1755) -> (7.1653, 42.05) construction
  line L286 (7.1653, 42.05) -> (7.6753, 43) construction
  line L287 (7.6753, 43) -> (7.1653, 43.95) construction
  line L288 (7.1653, 43.95) -> (7.1653, 46.8245) construction
  arc A240 (7.1653, 46.8245) -> (7.0189, 47.178) centre (6.6653, 46.8245) ccw construction
  line L289 (7.0189, 47.178) -> (3.0934, 51.1035) construction
  arc A241 (3.0934, 51.1035) -> (2.7398, 51.25) centre (2.7398, 50.75) ccw construction
  line L290 (2.7398, 51.25) -> (0.7572, 51.25) construction
  arc A242 (0.7572, 51.25) -> (0.2575, 50.7325) centre (0.7572, 50.75) ccw construction
  line L291 (0.2575, 50.7325) -> (0.2575, 47.5) construction
  arc A243 (-0.2425, 47) -> (0.2575, 47.5) centre (-0.2425, 47.5) ccw construction
  line L292 (-0.2425, 47) -> (-1.4999, 47) construction
  arc A244 (-1.9999, 47.5) -> (-1.4999, 47) centre (-1.4999, 47.5) ccw construction
  line L293 (-1.9999, 47.5) -> (-1.9999, 55.9999) construction
  arc A245 (0.0001, 57.9999) -> (-1.9999, 55.9999) centre (0.0001, 55.9999) ccw construction
  line L294 (0.0001, 57.9999) -> (8.5, 57.9999) construction
  arc A246 (9, 57.4999) -> (8.5, 57.9999) centre (8.5, 57.4999) ccw construction
  line L295 (9, 57.4999) -> (9, 56.2425) construction
  arc A247 (8.5, 55.7425) -> (9, 56.2425) centre (8.5, 56.2425) ccw construction
  line L296 (57.9999, 15.0099) -> (57.9999, 165.0067) construction
  line L297 (57.9999, 165.0067) -> (-1.9999, 165.0067)
  line L298 (-1.9999, 165.0067) -> (-1.9999, 14.9999)
  line L299 (-1.9999, 14.9999) -> (57.9999, 14.9999)
  line L300 (57.9999, 14.9999) -> (57.9999, 165.0067)
  circle A248 centre (13, 154.9529) radius 3.75
  circle A249 centre (13, 43) radius 3.75
  line L301 (13, 154.9529) -> (13, 43) construction
  line L302 (18.3247, 109.9529) -> (7.6753, 109.9529) construction
  circle A250 centre (13, 109.9529) radius 3.75
  point P0 (0, 0)
  dimension "d0" = 150.0068
  dimension "d1" = 59.9998
  dimension "d2" = 7.5
  measures "d0" distance of L297.end L298.end
  measures "d1" distance of L298.end L299.end
  measures "d2" diameter of A248
extrude "Plate1" add sketch "Sketch1" along normal blind 2
equation "\"BendRadius\" = Thickness"
equation "\"BendReliefWidth\" = Thickness"
equation "\"BendReliefDepth\" = 0.5 * Thickness"
equation "\"CornerReliefSize\" = 4 * Thickness"
equation "\"MinimumRemnant\" = 2 * Thickness"
equation "\"TransitionRadius\" = BendRadius"
equation "\"JacobiRadiusSize\" = BendRadius"
equation "\"GapSize\" = Thickness"
equation "\"d3\" = BendRadius"
equation "\"Thickness\" = 2"
body "Solid1"
